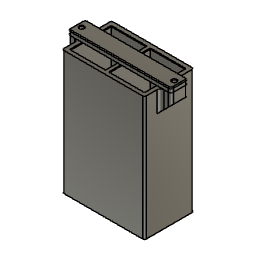
Battery Holder (Autodesk Fusion 360 design; units mm, degrees)
Autodesk Fusion 360 part; units mm, degrees
sketch "Battery" plane through (0, 0, 0) normal (0, 0, 1) x (1, 0, 0)
  line L0 (0, 0) -> (40, 0)
  line L1 (40, 0) -> (40, 47)
  line L2 (40, 47) -> (0, 47)
  line L3 (0, 47) -> (0, 0)
  line L4 (45, -0.2771) -> (85, -0.2771)
  line L5 (85, -0.2771) -> (85, 46.7229)
  line L6 (85, 46.7229) -> (45, 46.7229)
  line L7 (45, 46.7229) -> (45, -0.2771)
  dimension "d1" = 47
  dimension "d2" = 40
  dimension "d3" = 5
  constraint horizontal L0
  constraint vertical L1
  constraint horizontal L2
  constraint vertical L3
  constraint coincident L0.start L3.end
  constraint horizontal L4
  constraint vertical L5
  constraint horizontal L6
  constraint vertical L7
  constraint equal L3 L7
  constraint equal L0 L4
  measures "d1" distance of L0.start L2.end
  measures "d2" distance of L0.start L0.end
  measures "d3" horizontal distance of L0.end L4.start
extrude "Battery (1)" add sketch "Battery" along normal blind 138 makes body 1 at (0, 31.3333, 46) makes body 2 at (45, 31.0562, 46)
sketch "Base Box" plane through (0, 0, 0) normal (0, 0, -1) x (1, 0, 0)
  line L0 (0, 0) -> (0, -47)
  line L1 (0, -47) -> (40, -47)
  line L2 (40, -47) -> (40, 0)
  line L3 (40, 0) -> (0, 0)
  line L4 (-5, 5) -> (90, 5)
  line L5 (90, 5) -> (90, -52)
  line L6 (90, -52) -> (-5, -52)
  line L7 (-5, -52) -> (-5, 5)
  line L8 (85, 0.2771) -> (85, -46.7229)
  dimension "d6" = 5
  dimension "d7" = 5
  dimension "d8" = 5
  dimension "d9" = 5
  constraint horizontal L4
  constraint vertical L5
  constraint horizontal L6
  constraint vertical L7
  measures "d6" distance of L4.end L8
  measures "d7" horizontal distance of L0.start L4.start
  measures "d8" distance of L0.end L6
  measures "d9" distance of L0.start L4
extrude "Box Base" add sketch "Base Box" along normal blind 5 separate body contours L0 L1 L2 L3 | L4 L5 L6 L7 makes body 3
extrude "Extrude3" add 1 faces at (26.6667, 14, 0) along direction (0, 0, 1) up to surface (138 mm away) on bodies 3 bodies 3
combine "Combine1" operation cut target body 3 tool bodies 2 1 keep tools
ref_plane "WorkPlane1" through (42.5, 23.5, 66.5) normal (1, 0, 0) x (0, -1, 0)
sketch "Thumb Screw set" plane through (0, 0, 138) normal (0, 0, 1) x (-1, 0, 0)
  line L0 (0, -47) -> (-40, -47)
  line L1 (-40, -47) -> (-40, 0)
  line L2 (-40, 0) -> (0, 0)
  line L3 (0, 0) -> (0, -47)
  line L4 (-45, -46.7229) -> (-85, -46.7229)
  line L5 (-85, -46.7229) -> (-85, 0.2771)
  line L6 (-85, 0.2771) -> (-45, 0.2771)
  line L7 (-45, 0.2771) -> (-45, -46.7229)
  line L8 (-90, 5) -> (-90, -52)
  line L9 (-90, -52) -> (5, -52)
  line L10 (5, -52) -> (5, 5)
  line L11 (5, 5) -> (-90, 5)
  line L12 (-90, -13.5) -> (-102, -13.5)
  line L13 (-102, -13.5) -> (-102, -33.5)
  line L14 (-102, -33.5) -> (-90, -33.5)
  line L15 (-90, -33.5) -> (-90, -13.5)
  line L16 (-90, -33.5) -> (-90, -52) construction
  line L17 (-90, -13.5) -> (-90, 5) construction
  line L18 (-102, -23.5) -> (-90, -23.5) construction
  dimension "d20" = 12
  dimension "d30" = 20
  constraint horizontal L12
  constraint horizontal L14
  constraint vertical L15
  constraint coincident L8 L12.start
  constraint coincident L8.end L9.start
  constraint perpendicular L9 L16
  constraint coincident L8.start L11.end
  constraint perpendicular L11 L17
  constraint equal L16 L17
  constraint equal L12 L14
  constraint midpoint L13 L18.start
  constraint midpoint L15 L18.end
  measures "d20" distance of L12.start L12.end
  measures "d30" distance of L12.end L13.end
extrude "Thumb Screw set (1)" add sketch "Thumb Screw set" against normal blind 12 contours L8 L12 L13 L14 L15 bodies 3
chamfer "Chamfer1" distance 12 angle 45 1 edges at (90, 23.5, 126) on bodies 3
sketch "M4 screw/HS Clearance hole " plane through (0, 0, 138) normal (0, 0, 1) x (-1, 0, 0)
  line L0 (-90, -13.5) -> (-102, -13.5)
  line L1 (-102, -13.5) -> (-102, -33.5)
  line L2 (-102, -33.5) -> (-90, -33.5)
  circle A0 centre (-96, -23.5) radius 2
  circle A1 centre (-96, -23.5) radius 2.85
  line L3 (0, -47) -> (-40, -47)
  line L4 (-40, -47) -> (-40, 0)
  line L5 (-40, 0) -> (0, 0)
  line L6 (0, 0) -> (0, -47)
  line L7 (-45, -46.7229) -> (-85, -46.7229)
  line L8 (-85, -46.7229) -> (-85, 0.2771)
  line L9 (-85, 0.2771) -> (-45, 0.2771)
  line L10 (-45, 0.2771) -> (-45, -46.7229)
  line L11 (-90, -33.5) -> (-90, -52)
  line L12 (-90, -52) -> (5, -52)
  line L13 (5, -52) -> (5, 5)
  line L14 (5, 5) -> (-90, 5)
  line L15 (-90, 5) -> (-90, -13.5)
  line L16 (-102, -23.5) -> (-90, -23.5)
  dimension "d24" = 4
  dimension "d26" = 5.7
  constraint concentric A0 A1
  measures "d24" diameter of A0
  measures "d26" diameter of A1
extrude "Extrude5" cut sketch "M4 screw/HS Clearance hole " against normal through all contours A0 L16 | A0 L16 bodies 3
extrude "M4 HS Clearnace Hole" cut sketch "M4 screw/HS Clearance hole " against normal blind 8 contours A0 A1 L16 | A0 A1 L16 bodies 3
mirror "Mirror1" about plane through (42.5, 23.5, 66.5) normal (1, 0, 0) of bodies 3 merged
chamfer "Chamfer2" distance 0.6 angle 45 2 edges at (-13.6571, 22.4694, 138) (98.6571, 22.4694, 138) on bodies 3
chamfer "Chamfer3" distance 0.6 angle 45 8 edges at (0, 23.3615, 138) (20, 46.7229, 138) (40, 23.3615, 138) (20, 0, 138) (45, 23.3615, 138) (65, 46.7229, 138) (65, 0, 138) (85, 23.3615, 138) on bodies 3
fillet "Fillet1" radius 2 4 edges at (90, -5, 66.5) (90, 52, 66.5) (-5, -5, 66.5) (-5, 52, 66.5) on bodies 3
fillet "Fillet2" radius 3 4 edges at (102, 33.5, 132) (102, 13.5, 132) (-17, 33.5, 132) (-17, 13.5, 132) on bodies 3
fillet "Fillet3" radius 4 4 edges at (-5, 13.5, 126) (90, 13.5, 126) (90, 33.5, 126) (-5, 33.5, 126) on bodies 3
sketch "Tie Down" plane through (0, 0, 138) normal (0, 0, 1) x (-1, 0, 0)
  arc A0 (17, -16.5) -> (14, -13.5) centre (14, -16.5) ccw
  line L0 (14, -13.5) -> (9, -13.5)
  line L1 (-94, -13.5) -> (-99, -13.5)
  arc A1 (-99, -13.5) -> (-102, -16.5) centre (-99, -16.5) ccw
  line L2 (-102, -16.5) -> (-102, -30.5)
  arc A2 (-102, -30.5) -> (-99, -33.5) centre (-99, -30.5) ccw
  line L3 (-99, -33.5) -> (-94, -33.5)
  line L4 (9, -33.5) -> (14, -33.5)
  arc A3 (14, -33.5) -> (17, -30.5) centre (14, -30.5) ccw
  line L5 (17, -30.5) -> (17, -16.5)
  circle A4 centre (-96, -23.5) radius 3.45
  circle A5 centre (11, -23.5) radius 3.45
  line L6 (9, -33.5) -> (14, -33.5)
  line L7 (-99, -13.5) -> (-94, -13.5)
  arc A6 (17, -16.5) -> (14, -13.5) centre (14, -16.5) ccw
  circle A7 centre (11, -23.5) radius 2
  line L8 (17, -30.5) -> (17, -16.5)
  arc A8 (14, -33.5) -> (17, -30.5) centre (14, -30.5) ccw
  line L9 (14, -13.5) -> (9, -13.5)
  arc A9 (-99, -13.5) -> (-102, -16.5) centre (-99, -16.5) ccw
  arc A10 (-102, -30.5) -> (-99, -33.5) centre (-99, -30.5) ccw
  line L10 (-94, -33.5) -> (-99, -33.5)
  line L11 (-102, -30.5) -> (-102, -16.5)
  circle A11 centre (-96, -23.5) radius 2
  line L12 (9, -13.5) -> (-94, -13.5)
  line L13 (-94, -33.5) -> (9, -33.5)
  circle A12 centre (11, -23.5) radius 2.25
  circle A13 centre (-96, -23.5) radius 2.25
  dimension "d50" = 4.5
  constraint coincident L0.end L9.end
  constraint coincident L1.start L7.end
  constraint coincident L3.end L10.start
  constraint coincident L4.start L6.start
  constraint concentric A5 A12
  constraint concentric A11 A13
  constraint equal A12 A13
  measures "d50" diameter of A12
extrude "Extrude9" add sketch "Tie Down" along normal blind 5 separate body contours A0 L0 L1 A1 L2 A2 L3 L4 A3 L5 L6 L7 A6 L8 A8 L9 A9 A10 L10 L11 L12 L13 | A4 | A5 makes body 4
chamfer "Chamfer4" distance 0.6 angle 45 2 edges at (-8.9023, 22.6864, 143) (98.0977, 22.6864, 143) on bodies 4
fillet "Fillet4" radius 1 8 edges at (42.5, 13.5, 143) (101.1213, 14.3787, 143) (102, 23.5, 143) (101.1213, 32.6213, 143) (42.5, 33.5, 143) (-16.1213, 32.6213, 143) (-17, 23.5, 143) (-16.1213, 14.3787, 143) on bodies 4
hidden bodies 1 2
equation "d3 = BoxOffset"
equation "d6 = BoxOffset"
equation "d7 = BoxOffset"
equation "d8 = BoxOffset"
equation "d9 = BoxOffset"
equation "BoxOffset = 5 mm"
equation "M4_HSL_W = 5.7 mm" comment "Width of M4 HS"
equation "M4_HSL_L = 8 mm"
equation "d26 = M4_HSL_W"
equation "d27 = -M4_HSL_L"
equation "d32 = M4_HSL_W"
named bodies: "Battery 1", "Battery 2", "Box Base", "Tie Down"
